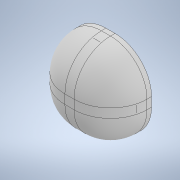
# Autodesk Inventor part: McCrea_horny_kos_walle_MIR2
Saved by Autodesk Inventor 2022 (Build 260153000, 153)
## iProperties
Created: 2022-02-08
Part Number: McCrea_horny_kos_walle_MIR2
Material: Generic
Document SubType Name: Modeling
Designer: Max
Density: 1 g/cm^3
Appearance: Default
Author: Max
Autodesk Inventor part; units mm, degrees
ref_plane "YZ Plane" through (0, 0, 0) normal (1, 0, 0) x (0, 1, 0)
ref_plane "XZ Plane" through (0, 0, 0) normal (0, 1, 0) x (-1, 0, 0)
ref_plane "XY Plane" through (0, 0, 0) normal (0, 0, 1) x (1, 0, 0)
sketch "Sketch1" plane through (0, 0, 0) normal (0, 0, 1) x (1, 0, 0)
  line L0 (-26.9068, 18.7438) -> (-8.9068, 18.7438)
  line L1 (-8.9068, 18.7438) -> (-8.9068, 0.7438)
  line L2 (-8.9068, 0.7438) -> (-26.9068, 0.7438)
  line L3 (-26.9068, 0.7438) -> (-26.9068, 18.7438)
  point P0 (0, 0)
  dimension "d5" = 18
  dimension "d6" = 18
  constraints: 8 end point, 2 parallel, 1 horizontal, 1 perpendicular
  measures "d5" distance of L0.end L1.end
  measures "d6" distance of L1.end L2.end
extrude "Extrusion1" add sketch "Sketch1" along normal blind 9
fillet "Fillet1" [suppressed]
fillet "Fillet2" radius 8 8 edges at (-17.9068, 18.7438, 9) (-8.9068, 18.7438, 4.5) (-8.9068, 9.7438, 9) (-17.9068, 0.7438, 9) (-26.9068, 9.7438, 9) (-26.9068, 0.7438, 4.5) (-26.9068, 18.7438, 4.5) (-8.9068, 0.7438, 4.5)
shell "Shell1" thickness 1 removed faces 1 at (-18.2401, 7.4105, 0)
sketch "Sketch2" plane through (0, 0, 0) normal (0, 0, -1) x (-1, 0, 0)
  line L0 (16.9068, 18.7438) -> (18.9068, 18.7438) projected
  arc A0 (26.9068, 10.7438) -> (18.9068, 18.7438) centre (18.9068, 10.7438) ccw projected
  arc A1 (25.9068, 10.7438) -> (18.9068, 17.7438) centre (18.9068, 10.7438) ccw projected
  line L1 (16.9068, 17.7438) -> (18.9068, 17.7438) projected
  arc A2 (16.9068, 17.7438) -> (9.9068, 10.7438) centre (16.9068, 10.7438) ccw projected
  arc A3 (16.9068, 18.7438) -> (8.9068, 10.7438) centre (16.9068, 10.7438) ccw projected
  line L2 (8.9068, 8.7438) -> (8.9068, 10.7438) projected
  line L3 (9.9068, 8.7438) -> (9.9068, 10.7438) projected
  arc A4 (8.9068, 8.7438) -> (16.9068, 0.7438) centre (16.9068, 8.7438) ccw projected
  arc A5 (9.9068, 8.7438) -> (16.9068, 1.7438) centre (16.9068, 8.7438) ccw projected
  line L4 (18.9068, 0.7438) -> (16.9068, 0.7438) projected
  line L5 (18.9068, 1.7438) -> (16.9068, 1.7438) projected
  arc A6 (18.9068, 0.7438) -> (26.9068, 8.7438) centre (18.9068, 8.7438) ccw projected
  arc A7 (18.9068, 1.7438) -> (25.9068, 8.7438) centre (18.9068, 8.7438) ccw projected
  line L6 (25.9068, 10.7438) -> (25.9068, 8.7438) projected
  line L7 (26.9068, 10.7438) -> (26.9068, 8.7438) projected
  line L8 (26.6568, 10.4938) -> (26.1568, 10.4938)
  line L9 (26.1568, 10.4938) -> (26.1568, 8.9938)
  line L10 (26.1568, 8.9938) -> (26.6568, 8.9938)
  line L11 (26.6568, 8.9938) -> (26.6568, 10.4938)
  circle A8 centre (17.9068, 9.7438) radius 8.75
  line L12 (17.1568, 17.9938) -> (18.6568, 17.9938)
  line L13 (18.6568, 17.9938) -> (18.6568, 18.4938)
  line L14 (18.6568, 18.4938) -> (17.1568, 18.4938)
  line L15 (17.1568, 18.4938) -> (17.1568, 17.9938)
  line L16 (9.6568, 8.9938) -> (9.6568, 10.4938)
  line L17 (9.6568, 10.4938) -> (9.1568, 10.4938)
  line L18 (9.1568, 10.4938) -> (9.1568, 8.9938)
  line L19 (9.1568, 8.9938) -> (9.6568, 8.9938)
  line L20 (18.6568, 1.4938) -> (17.1568, 1.4938)
  line L21 (17.1568, 1.4938) -> (17.1568, 0.9938)
  line L22 (17.1568, 0.9938) -> (18.6568, 0.9938)
  line L23 (18.6568, 0.9938) -> (18.6568, 1.4938)
  point P0 (0, 0)
  point P1 (18.6568, 18.4616)
  point P2 (17.1568, 18.4616)
  point P3 (9.189, 10.4938)
  point P4 (9.189, 8.9938)
  point P5 (17.1568, 1.026)
  point P6 (18.6568, 1.026)
  point P7 (26.6245, 8.9938)
  point P8 (26.6245, 10.4938)
  dimension "d12" = 1.5
  dimension "d13" = 0.5
  dimension "d14" = 0.25
  dimension "d16" = 0.25
  dimension "d18" = 8
  dimension "d19" = 17.5
  dimension "d22" = 360
  constraints: 32 end point, 2 parallel, 1 centre point, 1 horizontal, 1 perpendicular, 33 other
  measures "d12" distance of L8.end L9.end
  measures "d13" distance of L8.start L8.end
  measures "d14" distance between parallel lines of L7 L11
  measures "d16" distance from line of A0.centre L8
  measures "d18" radius of A6
  measures "d19" diameter of A8
extrude "Extrusion2" cut sketch "Sketch2" against normal blind 3 contours L13 L12 L15 A8
extrude "Extrusion3" cut sketch "Sketch2" against normal blind 3 contours A8 L10 L9 L8 | A8 L21 L20 L23 | L17 L16 L19 A8
body "Solid1"
